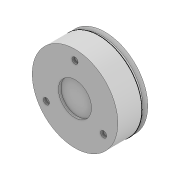
# Autodesk Inventor part: sensor
Saved by Autodesk Inventor 2020 (Build 240168000, 168)
## iProperties
Created: 2020-08-31
Part Number: sensor
Material: 일반
Document SubType Name: Modeling
Designer: 이호석
Mass: 92.172 g
Surface Area: 135.353 cm^2
Volume: 92.172 cm^3
Density: 1 g/cm^3
Appearance: 기본값
Author: 이호석
Autodesk Inventor part; units mm, degrees
ref_plane "YZ Plane" through (0, 0, 0) normal (1, 0, 0) x (0, 1, 0)
ref_plane "XZ Plane" through (0, 0, 0) normal (0, 1, 0) x (-1, 0, 0)
ref_plane "XY Plane" through (0, 0, 0) normal (0, 0, 1) x (1, 0, 0)
sketch "스케치1" plane through (0, 0, 0) normal (0, 0, 1) x (1, 0, 0)
  circle A0 centre (0, 0) radius 35
  dimension "d0" = 70
  constraints: 1 centre point, 1 coincident
  measures "d0" diameter of A0
extrude "돌출1" add sketch "스케치1" along normal blind 19.5
sketch "스케치2" plane through (0, 0, 19.5) normal (0, 0, 1) x (1, 0, 0)
  line L0 (0, 0) -> (0, 27)
  circle A0 centre (0, 27) radius 2.5
  circle A1 centre (0, 0) radius 35 projected
  circle A2 centre (-23.3827, -13.5) radius 2.5
  circle A3 centre (23.3827, -13.5) radius 2.5
  circle A4 centre (0, 0) radius 13.5
  dimension "d3" = 27
  dimension "d4" = 5
  dimension "d7" = 360
  constraints: 4 centre point, 2 coincident, 2 end point, 1 vertical, 7 other
  measures "d3" distance of L0.start L0.end
  measures "d4" diameter of A0
extrude "돌출2" cut sketch "스케치2" against normal blind 2 contours A0 | A2 | A3 | A4
sketch "스케치3" plane through (0, 0, 0) normal (0, 0, -1) x (-1, 0, 0)
  circle A0 centre (0, 0) radius 35
  constraints: 1 centre point, 1 coincident
ref_plane "작업 평면1" through (0, 0, -2.5) normal (0, 0, -1) x (-1, 0, 0)
sketch "스케치4" plane through (0, 0, -2.5) normal (0, 0, -1) x (-1, 0, 0)
  circle A0 centre (0, 0) radius 33.5
  dimension "d12" = 67
  constraints: 1 centre point, 1 coincident
  measures "d12" diameter of A0
loft "로프트1" add profiles "스케치4" section 1 edges at (-35, 0, 0)
ref_plane "작업 평면2" through (0, 0, -5) normal (0, 0, -1) x (-1, 0, 0)
sketch "스케치5" plane through (0, 0, -5) normal (0, 0, -1) x (-1, 0, 0)
  circle A0 centre (0, 0) radius 35
  dimension "d18" = 70
  constraints: 1 centre point, 1 coincident
  measures "d18" diameter of A0
loft "로프트2" add profiles "스케치5" section 1 edges at (-33.5, 0, -2.5)
sketch "스케치6" plane through (0, 0, -5) normal (0, 0, -1) x (-1, 0, 0)
  circle A0 centre (0, 0) radius 2.5
  dimension "d23" = 5
  constraints: 1 centre point, 1 coincident
  measures "d23" diameter of A0
extrude "돌출3" cut sketch "스케치6" against normal blind 2
